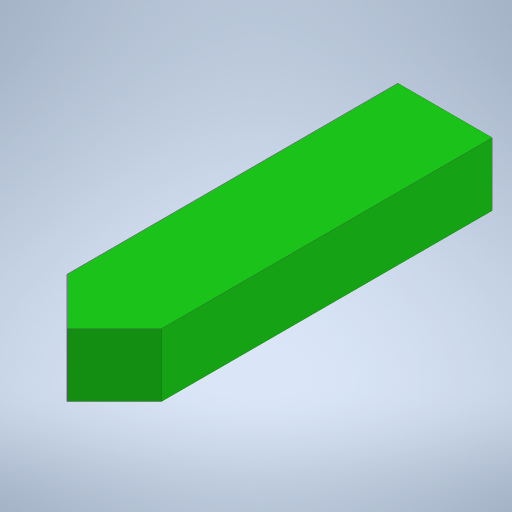
# Autodesk Inventor part: PEÇA MOVEL
Saved by Autodesk Inventor 2023 (Build 270158000, 158)
## iProperties
Created: 2023-10-18
Part Number: PEÇA MOVEL
Material: Genérico
Document SubType Name: Modeling
Designer: vinicius.sena
Density: 1 g/cm^3
Appearance: Padrão
Author: vinicius.sena
Autodesk Inventor part; units mm, degrees
ref_plane "YZ Plane" through (0, 0, 0) normal (1, 0, 0) x (0, 1, 0)
ref_plane "XZ Plane" through (0, 0, 0) normal (0, 1, 0) x (-1, 0, 0)
ref_plane "XY Plane" through (0, 0, 0) normal (0, 0, 1) x (1, 0, 0)
sketch "Esboço1" plane through (0, 0, 0) normal (0, 0, 1) x (1, 0, 0)
  line L0 (-3, 2) -> (3, 2)
  line L1 (3, 2) -> (3, -2)
  line L2 (3, -2) -> (-3, -2)
  line L3 (-3, -2) -> (-3, 2)
  line L4 (-3, 2) -> (3, -2) construction
  line L5 (3, 2) -> (-3, -2) construction
  point P0 (0, 0)
  dimension "d0" = 6
  dimension "d1" = 4
  constraints: 12 end point, 2 midpoint, 2 parallel, 1 horizontal, 1 perpendicular
  measures "d0" distance of L1.end L2.end
  measures "d1" distance of L0.end L1.end
extrude "Extrusão1" add sketch "Esboço1" along normal blind 24
chamfer "Chanfro1" distance 3 angle 45 2 edges at (3, 0, 24) (-3, 0, 24)
